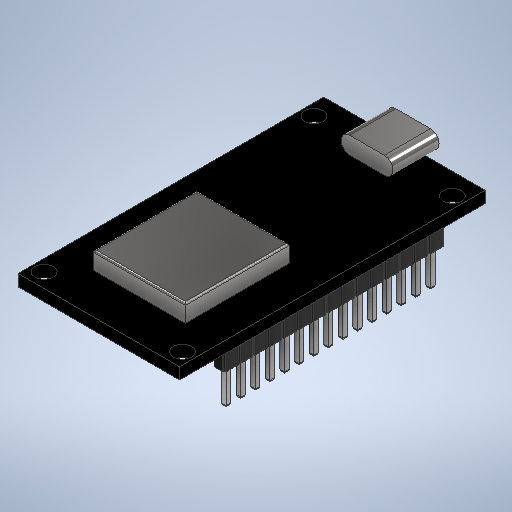
# Autodesk Inventor part: ESP32_DevBoard
Saved by Autodesk Inventor 2025.1 (Build 291241020, 241B)
## iProperties
Created: 2024-08-30
Part Number: ESP32_DevBoard
Material: Generic
Document SubType Name: Modeling
Designer: andre
Density: 1 g/cm^3
Appearance: Default
Author: andre
Autodesk Inventor part; units mm, degrees
ref_plane "YZ Plane" through (0, 0, 0) normal (1, 0, 0) x (0, 1, 0)
sketch "Sketch1" plane through (0, 0, 0) normal (0, 1, 0) x (-1, 0, 0)
  line L0 (0, 0) -> (28, 0)
  line L1 (28, 0) -> (28, -53)
  line L2 (28, -53) -> (0, -53)
  line L3 (0, -53) -> (0, 0)
  dimension "d0" = 53
  dimension "d1" = 28
  constraints: 8 end point, 2 parallel, 1 horizontal, 1 perpendicular
  measures "d0" distance of L0.end L1.end
  measures "d1" distance of L1.end L2.end
extrude "Extrusion1" add sketch "Sketch1" along normal blind 2
sketch "Sketch2" plane through (0, 2, 0) normal (0, 1, 0) x (1, 0, 0)
  line L0 (0, 53) -> (-28, 53) projected
  line L1 (-28, 53) -> (-28, 0) projected
  line L2 (-28, 0) -> (0, 0) projected
  line L3 (0, 0) -> (0, 53) projected
  line L4 (-22, 25) -> (-6, 25)
  line L5 (-6, 25) -> (-6, 7)
  line L6 (-6, 7) -> (-22, 7)
  line L7 (-22, 7) -> (-22, 25)
  point P0 (-14, 7)
  point P1 (-14, 0)
  dimension "d4" = 16
  dimension "d5" = 18
  dimension "d6" = 7
  constraints: 8 end point, 2 midpoint, 2 parallel, 1 horizontal, 1 perpendicular, 1 vertical alignment
  measures "d4" distance of L5.end L6.end
  measures "d5" distance of L4.end L5.end
  measures "d6" distance between parallel lines of L2 L6
extrude "Extrusion2" add sketch "Sketch2" along normal blind 3 contours L4 L5 L6 L7
fillet "Fillet1" radius 0.3 4 edges at (-14, 5, -7) (-6, 5, -16) (-22, 5, -16) (-14, 5, -25)
sketch "Sketch3" plane through (0, 0, -53) normal (0, 0, -1) x (-1, 0, 0)
  line L0 (0, 0) -> (28, 0) projected
  line L1 (28, 0) -> (28, 2) projected
  line L2 (0, 2) -> (28, 2) projected
  line L3 (0, 0) -> (0, 2) projected
  arc A0 (11, 5) -> (11, 2) centre (11, 3.5) ccw
  arc A1 (17, 2) -> (17, 5) centre (17, 3.5) ccw
  line L4 (11, 5) -> (17, 5)
  line L5 (17, 2) -> (11, 2)
  line L6 (18.5, 12.8839) -> (18.5, 7.7714) construction
  line L7 (9.5, 12.1713) -> (9.5, 6.1147) construction
  arc A2 (17, 2.33) -> (17, 4.67) centre (17, 3.5) ccw
  line L8 (17, 2.33) -> (11, 2.33)
  arc A3 (11, 4.67) -> (11, 2.33) centre (11, 3.5) ccw
  line L9 (11, 4.67) -> (17, 4.67)
  point P0 (14, 4.67)
  point P1 (14, 2)
  dimension "d10" = 9
  dimension "d11" = 3
  dimension "d12" = 0.33
  constraints: 12 end point, 8 point on circle, 6 tangent, 4 centre point, 2 horizontal, 2 midpoint, 2 vertical, 1 horizontal alignment, 1 vertical alignment, 3 other
  measures "d10" distance between parallel lines of L6 L7
  measures "d11" distance between parallel lines of L5 L4
  measures "d12" distance between parallel lines of L4 L9
extrude "Extrusion3" add sketch "Sketch3" along normal blind 1.5 and the other way blind 6.5 contours A0 L4 A1 L2
sketch "Sketch5" plane through (0, 2, 0) normal (0, 1, 0) x (1, 0, 0)
  circle A0 centre (-2, 2.5) radius 1.6
  circle A1 centre (-26, 2.5) radius 1.6
  circle A2 centre (-26, 49.3) radius 1.6
  circle A3 centre (-2, 49.3) radius 1.6
  line L0 (-7.0467, 0.9) -> (-3.7447, 0.9) construction
  line L1 (-6.7299, 50.9) -> (-3.3876, 50.9) construction
  line L2 (-2, 49.3) -> (-2, 2.5) construction
  line L3 (-6, 25) -> (-6, 7) construction
  line L4 (-11, 46.5) -> (-11, 53) construction
  line L5 (-17, 46.5) -> (-17, 53) construction
  line L6 (-17, 53) -> (-28, 53) construction
  line L7 (-28, 53) -> (-28, 0) construction
  line L8 (-28, 0) -> (0, 0) construction
  line L9 (0, 0) -> (0, 53) construction
  line L10 (0, 53) -> (-11, 53) construction
  line L11 (-22, 7) -> (-22, 25) construction
  line L12 (-22, 25) -> (-6, 25) construction
  line L13 (-6, 25) -> (-6, 7) construction
  line L14 (-6, 7) -> (-22, 7) construction
  line L15 (-0.4, 0.8278) -> (-0.4, 6.2896) construction
  line L16 (-27.6, 1.6648) -> (-27.6, 8.2425) construction
  line L17 (-27.6, 4.9536) -> (-0.4, 4.9536) construction
  line L18 (-11, 46.5) -> (-17, 46.5) projected
  point P0 (-5.0588, 50.9)
  point P1 (0, 26.5)
  point P2 (-2, 25.9)
  point P3 (-14, 0)
  point P4 (-14, 4.9536)
  point P5 (-22, 16)
  dimension "d17" = 3.2
  dimension "d18" = 3.2
  dimension "d19" = 3.2
  dimension "d20" = 3.2
  dimension "d21" = 50
  dimension "d69" = 4
  dimension "d70" = 4.5
  dimension "d72" = 4
  constraints: 12 end point, 7 midpoint, 4 centre point, 4 tangent, 3 horizontal, 2 horizontal alignment, 2 vertical, 1 parallel, 1 point on line, 1 vertical alignment
  measures "d17" diameter of A0
  measures "d18" diameter of A1
  measures "d19" diameter of A2
  measures "d20" diameter of A3
  measures "d21" distance from line of L0 point (-5.059, 50.9)
  measures "d69" horizontal distance of A1.centre point (-22, 16)
  measures "d70" distance from line of A1.centre L14
  measures "d72" distance from line of L2.end L13
extrude "Extrusion5" cut sketch "Sketch5" against normal through all
sketch "Sketch6" plane through (0, 0, 0) normal (0, -1, 0) x (1, 0, 0)
  line L0 (-27.8, -46) -> (-25.8, -46)
  line L1 (-25.8, -46) -> (-25.8, -8)
  line L2 (-25.8, -8) -> (-27.8, -8)
  line L3 (-27.8, -8) -> (-27.8, -46)
  line L4 (-28, -53) -> (-28, 0) projected
  line L5 (-28, 0) -> (0, 0) projected
  dimension "d30" = 2
  dimension "d31" = 38
  dimension "d32" = 0.2
  dimension "d33" = 8
  constraints: 8 end point, 2 parallel, 1 horizontal, 1 perpendicular
  measures "d30" distance of L2.end L1.end
  measures "d31" distance of L1.end L0.end
  measures "d32" distance between parallel lines of L4 L3
  measures "d33" distance between parallel lines of L5 L2
extrude "Extrusion6" add sketch "Sketch6" along normal blind 3
ref_plane "Work Plane1" through (-14, 0, -53) normal (1, 0, 0) x (0, 0, -1)
sketch "Sketch9" plane through (0, 0, -46.5) normal (0, 0, 1) x (1, 0, 0)
  arc A0 (-11, 2) -> (-11, 5) centre (-11, 3.5) ccw projected
  line L0 (-11, 5) -> (-17, 5) projected
  arc A1 (-17, 5) -> (-17, 2) centre (-17, 3.5) ccw projected
  line L1 (-11, 2) -> (-17, 2) projected
  line L2 (-17, 4.67) -> (-11, 4.67) projected
  arc A2 (-11, 2.33) -> (-11, 4.67) centre (-11, 3.5) ccw projected
  line L3 (-11, 2.33) -> (-17, 2.33) projected
  arc A3 (-17, 4.67) -> (-17, 2.33) centre (-17, 3.5) ccw projected
  point P0 (0, 0)
extrude "Extrusion7" add sketch "Sketch9" against normal blind 1 contours L2 A2 L3 A3
sketch "Sketch10" plane through (0, -3, 0) normal (0, -1, 0) x (1, 0, 0)
  line L0 (-25.8, -46) -> (-25.8, -8) projected
  line L1 (-25.8, -8) -> (-27.8, -8) projected
  line L2 (-27.8, -8) -> (-27.8, -46) projected
  line L3 (-27.8, -46) -> (-25.8, -46) projected
  line L4 (-27.2, -45.1) -> (-26.4, -45.1)
  line L5 (-26.4, -45.1) -> (-26.4, -44.3)
  line L6 (-26.4, -44.3) -> (-27.2, -44.3)
  line L7 (-27.2, -44.3) -> (-27.2, -45.1)
  point P0 (0, 0)
  point P1 (-26.8, -45.1)
  point P2 (-26.8, -46)
  dimension "d40" = 0.8
  dimension "d41" = 0.8
  dimension "d42" = 0.9
  constraints: 8 end point, 2 midpoint, 2 parallel, 1 horizontal, 1 perpendicular, 1 vertical alignment
  measures "d40" distance of L6.end L4.start
  measures "d41" distance of L5.end L6.end
  measures "d42" distance between parallel lines of L3 L4
extrude "Extrusion8" add sketch "Sketch10" along normal blind 6 contours L7 L6 L5 L4
chamfer "Chamfer1" distance 0.1 distance2 0.3 4 edges at (-26.4, -9, -44.7) (-26.8, -9, -45.1) (-26.8, -9, -44.3) (-27.2, -9, -44.7) measured on face at (-26.8, -9, -44.6) measured on face at (-26.7, -9, -44.7) measured on face at (-26.8, -9, -44.8) measured on face at (-26.9, -9, -44.7)
fillet "Fillet2" radius 0.1 4 edges at (-26.8, -9, -45) (-26.5, -9, -44.7) (-26.8, -9, -44.4) (-27.1, -9, -44.7)
pattern_linear "Rectangular Pattern1" count 15 spacing 2.53 along (0, 0, 1) of "Extrusion8", "Fillet2", "Chamfer1"
sketch "Sketch11" plane through (0, -3, 0) normal (0, -1, 0) x (1, 0, 0)
  line L0 (-26.4, -9.68) -> (-27.2, -9.68) projected
  line L1 (-27.2, -9.68) -> (-27.2, -8.88) projected
  line L2 (-27.2, -8.88) -> (-26.4, -8.88) projected
  line L3 (-26.4, -8.88) -> (-26.4, -9.68) projected
  line L4 (-26.4, -12.21) -> (-27.2, -12.21) projected
  line L5 (-27.2, -12.21) -> (-27.2, -11.41) projected
  line L6 (-27.2, -11.41) -> (-26.4, -11.41) projected
  line L7 (-26.4, -11.41) -> (-26.4, -12.21) projected
  line L8 (-26.4, -14.74) -> (-27.2, -14.74) projected
  line L9 (-27.2, -14.74) -> (-27.2, -13.94) projected
  line L10 (-27.2, -13.94) -> (-26.4, -13.94) projected
  line L11 (-26.4, -13.94) -> (-26.4, -14.74) projected
  line L12 (-26.4, -17.27) -> (-27.2, -17.27) projected
  line L13 (-27.2, -17.27) -> (-27.2, -16.47) projected
  line L14 (-27.2, -16.47) -> (-26.4, -16.47) projected
  line L15 (-26.4, -16.47) -> (-26.4, -17.27) projected
  line L16 (-26.4, -19.8) -> (-27.2, -19.8) projected
  line L17 (-27.2, -19.8) -> (-27.2, -19) projected
  line L18 (-27.2, -19) -> (-26.4, -19) projected
  line L19 (-26.4, -19) -> (-26.4, -19.8) projected
  line L20 (-26.4, -22.33) -> (-27.2, -22.33) projected
  line L21 (-27.2, -22.33) -> (-27.2, -21.53) projected
  line L22 (-27.2, -21.53) -> (-26.4, -21.53) projected
  line L23 (-26.4, -21.53) -> (-26.4, -22.33) projected
  line L24 (-26.4, -24.86) -> (-27.2, -24.86) projected
  line L25 (-27.2, -24.86) -> (-27.2, -24.06) projected
  line L26 (-27.2, -24.06) -> (-26.4, -24.06) projected
  line L27 (-26.4, -24.06) -> (-26.4, -24.86) projected
  line L28 (-26.4, -27.39) -> (-27.2, -27.39) projected
  line L29 (-27.2, -27.39) -> (-27.2, -26.59) projected
  line L30 (-27.2, -26.59) -> (-26.4, -26.59) projected
  line L31 (-26.4, -26.59) -> (-26.4, -27.39) projected
  line L32 (-26.4, -29.92) -> (-27.2, -29.92) projected
  line L33 (-27.2, -29.92) -> (-27.2, -29.12) projected
  line L34 (-27.2, -29.12) -> (-26.4, -29.12) projected
  line L35 (-26.4, -29.12) -> (-26.4, -29.92) projected
  line L36 (-26.4, -32.45) -> (-27.2, -32.45) projected
  line L37 (-27.2, -32.45) -> (-27.2, -31.65) projected
  line L38 (-27.2, -31.65) -> (-26.4, -31.65) projected
  line L39 (-26.4, -31.65) -> (-26.4, -32.45) projected
  line L40 (-26.4, -34.98) -> (-27.2, -34.98) projected
  line L41 (-27.2, -34.98) -> (-27.2, -34.18) projected
  line L42 (-27.2, -34.18) -> (-26.4, -34.18) projected
  line L43 (-26.4, -34.18) -> (-26.4, -34.98) projected
  line L44 (-26.4, -37.51) -> (-27.2, -37.51) projected
  line L45 (-27.2, -37.51) -> (-27.2, -36.71) projected
  line L46 (-27.2, -36.71) -> (-26.4, -36.71) projected
  line L47 (-26.4, -36.71) -> (-26.4, -37.51) projected
  line L48 (-26.4, -40.04) -> (-27.2, -40.04) projected
  line L49 (-27.2, -40.04) -> (-27.2, -39.24) projected
  line L50 (-27.2, -39.24) -> (-26.4, -39.24) projected
  line L51 (-26.4, -39.24) -> (-26.4, -40.04) projected
  line L52 (-26.4, -42.57) -> (-27.2, -42.57) projected
  line L53 (-27.2, -42.57) -> (-27.2, -41.77) projected
  line L54 (-27.2, -41.77) -> (-26.4, -41.77) projected
  line L55 (-26.4, -41.77) -> (-26.4, -42.57) projected
  line L56 (-26.4, -45.1) -> (-27.2, -45.1) projected
  line L57 (-27.2, -45.1) -> (-27.2, -44.3) projected
  line L58 (-27.2, -44.3) -> (-26.4, -44.3) projected
  line L59 (-26.4, -44.3) -> (-26.4, -45.1) projected
  line L60 (-25.8, -46) -> (-25.8, -8) projected
  line L61 (-25.8, -8) -> (-27.8, -8) projected
  line L62 (-27.8, -8) -> (-27.8, -46) projected
  line L63 (-27.8, -46) -> (-25.8, -46) projected
  line L64 (-26.5721, -44.4721) -> (-26.5721, -44.9279) construction
  line L65 (-27.0279, -44.4721) -> (-26.5721, -44.4721) construction
  line L66 (-27.0279, -44.9279) -> (-27.0279, -44.4721) construction
  line L67 (-26.5721, -44.9279) -> (-27.0279, -44.9279) construction
  line L68 (-26.5721, -41.9421) -> (-26.5721, -42.3979) construction
  line L69 (-27.0279, -41.9421) -> (-26.5721, -41.9421) construction
  line L70 (-27.0279, -42.3979) -> (-27.0279, -41.9421) construction
  line L71 (-26.5721, -42.3979) -> (-27.0279, -42.3979) construction
  line L72 (-27.0279, -44.7) -> (-27.8, -43.435) construction
  line L73 (-27.0279, -42.17) -> (-27.8, -43.435) construction
  line L74 (-27.0279, -44.9279) -> (-27.0279, -44.4721) construction
  line L75 (-27.0279, -42.3979) -> (-27.0279, -41.9421) construction
  line L76 (-27.8, -43.635) -> (-27.57, -43.5397)
  arc A0 (-27.57, -43.5397) -> (-27.57, -43.3303) centre (-27.6133, -43.435) ccw
  line L77 (-27.57, -43.3303) -> (-27.8, -43.235)
  point P0 (0, 0)
  point P1 (-27.5, -43.435)
  dimension "d52" = 0.3
  dimension "d53" = 0.4
  dimension "d54" = 45
  constraints: 8 end point, 3 point on circle, 3 point on line, 2 equal length, 2 midpoint, 2 tangent, 1 centre point, 1 horizontal alignment
  measures "d52" distance from line of L62 point (-27.5, -43.435)
  measures "d53" distance of L77.end L76.start
  measures "d54" angle of L77 L76
extrude "Extrusion9" cut sketch "Sketch11" against normal up to surface (3 mm away) contours L62 L77 A0 L76
ref_plane "Work Plane3" through (-26.8, -3, -46) normal (-1, 0, 0) x (0, 0, 1)
mirror "Mirror2" about plane through (-26.8, -3, -46) normal (-1, 0, 0) of "Extrusion9"
pattern_linear "Rectangular Pattern2" count 15 spacing 2.53 along (0, 0, 1) of "Extrusion9", "Mirror2"
pattern_linear "Rectangular Pattern3" count 2 spacing 2.53 along (0, 0, -1) of "Extrusion9", "Mirror2"
mirror "Mirror3" about plane through (-14, 0, -53) normal (1, 0, 0) of "Extrusion6", "Extrusion8", "Fillet2", "Chamfer1", "Rectangular Pattern1", "Extrusion9", "Mirror2", "Rectangular Pattern2"
sketch "Sketch12" plane through (0, 2, 0) normal (0, 1, 0) x (1, 0, 0)
  circle A0 centre (-26, 2.5) radius 1.6 projected
  circle A1 centre (-26, 49.3) radius 1.6 projected
  circle A2 centre (-2, 2.5) radius 1.6 projected
  circle A3 centre (-2, 49.3) radius 1.6 projected
  line L0 (-17, 46.5) -> (-17, 53) projected
  line L1 (-17, 53) -> (-28, 53) projected
  line L2 (-28, 53) -> (-28, 0) projected
  line L3 (-28, 0) -> (0, 0) projected
  line L4 (0, 0) -> (0, 53) projected
  line L5 (0, 53) -> (-11, 53) projected
  line L6 (-11, 46.5) -> (-11, 53) projected
  line L7 (-11, 46.5) -> (-17, 46.5) projected
  line L8 (-22, 7) -> (-22, 25) projected
  line L9 (-22, 25) -> (-6, 25) projected
  line L10 (-6, 25) -> (-6, 7) projected
  line L11 (-6, 7) -> (-22, 7) projected
  line L12 (-22, 7) -> (-6, 25) construction
  line L13 (-22, 25) -> (-6, 7) construction
  line L14 (-11, 46.5) -> (-9.5, 46.5) construction
  line L15 (-18.5, 46.5) -> (-17, 46.5) construction
  line L16 (-11, 46.5) -> (-17, 46.5) construction
  point P0 (-14, 16)
  point P1 (-14, 16)
  point P2 (-10.25, 46.5)
  point P3 (-17.75, 46.5)
  point P4 (-14, 46.5)
  dimension "d63" = 14
  dimension "d64" = 16
  dimension "d65" = 7.5
  dimension "d66" = 6.5
  dimension "d67" = 53
  dimension "d68" = 28
  constraints: 5 midpoint, 4 end point
  measures "d63" distance from line of L2 point (-14, 16)
  measures "d64" distance from line of L3 point (-14, 16)
  measures "d65" distance of point (-10.25, 46.5) point (-17.75, 46.5)
  measures "d66" distance from line of point (-14, 46.5) L1
  measures "d67" distance between parallel lines of L3 L5
  measures "d68" distance between parallel lines of L2 L4
ref_plane "Work Plane4" through (-14, 0, -53) normal (1, 0, 0) x (0, 0, -1)
body "Solid1"
